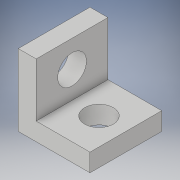
# Autodesk Inventor part: 0.5 L-Bracket
Saved by Autodesk Inventor 2019 (Build 230136000, 136)
## iProperties
Created: 2018-11-11
Part Number: 0.5 L-Bracket
Material: Generic
Document SubType Name: Modeling
Designer: maste
Density: 1 g/cm^3
Appearance: Default
Author: maste
Autodesk Inventor part; units mm, degrees
ref_plane "YZ Plane" through (0, 0, 0) normal (1, 0, 0) x (0, 1, 0)
ref_plane "XZ Plane" through (0, 0, 0) normal (0, 1, 0) x (-1, 0, 0)
ref_plane "XY Plane" through (0, 0, 0) normal (0, 0, 1) x (1, 0, 0)
sketch "Sketch1" plane through (0, 0, 0) normal (0, 0, 1) x (1, 0, 0)
  line L0 (0, 0) -> (3.175, 0)
  line L1 (3.175, 0) -> (3.175, 12.7)
  line L2 (3.175, 12.7) -> (0, 12.7)
  line L3 (0, 12.7) -> (0, 0)
  line L4 (0, 0) -> (12.7, 0)
  line L5 (12.7, 0) -> (12.7, 3.175)
  line L6 (12.7, 3.175) -> (0, 3.175)
  line L7 (0, 3.175) -> (0, 0)
  dimension "d0" = 3.175
  dimension "d1" = 12.7
  dimension "d2" = 12.7
  dimension "d3" = 3.175
  constraints: 16 end point, 4 parallel, 2 horizontal, 2 perpendicular
  measures "d0" distance of L2.end L1.end
  measures "d1" distance of L0.end L1.end
  measures "d2" distance of L6.end L5.end
  measures "d3" distance of L5.end L4.end
extrude "Extrusion1" add sketch "Sketch1" along normal blind 12.7
sketch "Sketch2" plane through (3.175, 3.175, 0) normal (0, 1, 0) x (1, 0, 0)
  line L0 (-3.175, 0) -> (-3.175, -12.7) projected
  line L1 (-3.175, 0) -> (9.525, 0) projected
  line L2 (9.525, 0) -> (0, -12.7)
  line L3 (0, -12.7) -> (0, 0)
  line L4 (9.525, 0) -> (9.525, -12.7) projected
  line L5 (0, 0) -> (9.525, -12.7)
  circle A0 centre (4.7625, -6.35) radius 2.54
  dimension "d8" = 5.08
  constraints: 6 end point, 1 centre point, 1 midpoint, 1 point on line, 1 vertical
  measures "d8" diameter of A0
extrude "Extrusion2" cut sketch "Sketch2" against normal blind 12.7 contours A0 L2 L5 | L5 L2 A0 | A0 L5 L2 | L2 L5 A0
sketch "Sketch3" plane through (3.175, 3.175, 0) normal (1, 0, 0) x (0, 0, -1)
  line L0 (0, 9.525) -> (-12.7, 9.525) projected
  line L1 (-12.7, 9.525) -> (0, 0)
  line L2 (0, 9.525) -> (-12.7, 0)
  circle A0 centre (-6.35, 4.7625) radius 2.54
  point P0 (0, -3.175)
  dimension "d11" = 5.08
  constraints: 4 end point, 1 centre point, 1 midpoint
  measures "d11" diameter of A0
extrude "Extrusion3" cut sketch "Sketch3" against normal blind 12.7 contours A0 L1 L2 | L2 L1 A0 | L1 L2 A0 | L1 A0 L2
body "Solid1"
